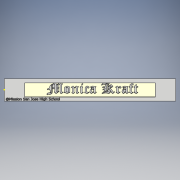
# Autodesk Inventor part: NameTag
Saved by Autodesk Inventor 2018 (Build 220112000, 112)
## iProperties
Created: 2019-03-18
Part Number: NameTag
Material: Generic
Document SubType Name: Modeling
Designer: This kid
Density: 1 g/cm^3
Appearance: Default
Author: This kid
Autodesk Inventor part; units mm, degrees
(part 1 of 3)
ref_plane "YZ Plane" through (0, 0, 0) normal (1, 0, 0) x (0, 1, 0)
ref_plane "XZ Plane" through (0, 0, 0) normal (0, 1, 0) x (-1, 0, 0)
ref_plane "XY Plane" through (0, 0, 0) normal (0, 0, 1) x (1, 0, 0)
sketch "Sketch1" plane through (0, 0, 0) normal (0, 0, 1) x (1, 0, 0)
  line L0 (0, 6.6514) -> (5.7603, -3.3257)
  line L1 (5.7603, -3.3257) -> (-5.7603, -3.3257)
  line L2 (-5.7603, -3.3257) -> (0, 6.6514)
  point P0 (0, 0)
  point P1 (0, 0)
  constraints: 6 end point, 1 coincident, 7 other
extrude "Extrusion1" add sketch "Sketch1" along normal blind 76.2
sketch "Sketch2" plane through (-5.7603, -3.3257, 0) normal (-0.8660254, 0.5, 0) x (0, 0, 1)
  line L0 (9.0292, 2.0917) -> (67.1704, 2.0917)
  line L1 (67.1704, 2.0917) -> (67.1704, 9.2481)
  line L2 (67.1704, 9.2481) -> (9.0292, 9.2481)
  line L3 (9.0292, 9.2481) -> (9.0292, 2.0917)
  line L4 (0, 5.7603) -> (9.0292, 5.6699) construction
  line L5 (67.1704, 5.7603) -> (76.2, 5.7603) construction
  constraints: 12 end point, 2 parallel, 1 equal length, 1 horizontal, 1 midpoint, 1 perpendicular, 1 point on line
extrude "Extrusion2" add sketch "Sketch2" along normal blind 0.2286
sketch "Sketch3" plane through (-5.9582, -3.2114, 0) normal (-0.8660254, 0.5, 0) x (0, 0, 1)
  point P0 (0, 5.7603)
sketch "Sketch4" plane through (-5.9582, -3.2114, 0) normal (-0.8660254, 0.5, 0) x (0, 0, 1)
  line L0 (9.8332, 9.129) -> (68.5929, 9.129) construction
  line L1 (68.5929, 9.129) -> (68.5929, 1.5104) construction
  line L2 (68.5929, 1.5104) -> (9.8332, 1.5104) construction
  line L3 (9.8332, 1.5104) -> (9.8332, 9.129) construction
  line L4 (25.7804, 8.8183) -> (25.8898, 8.7045)
  spline S0 degree 2 poles (25.8898, 8.7045) (25.6535, 8.442) (25.5222, 8.1094) (25.5222, 7.7724) knots 0 0 0 1 2 2 2
  line L5 (25.5222, 7.7724) -> (25.5222, 4.9936)
  spline S1 degree 2 poles (25.5222, 4.9936) (25.5222, 4.5647) (25.6666, 4.3459) (25.7848, 4.3459) knots 0 0 0 1 2 2 2
  spline S2 degree 2 poles (25.7848, 4.3459) (25.8854, 4.3459) (26.0692, 4.5122) knots 0 0 0 1 1 1
  line L6 (26.0692, 4.5122) -> (26.1743, 4.3721)
  line L7 (26.1743, 4.3721) -> (25.3034, 3.6895)
  spline S3 degree 2 poles (25.3034, 3.6895) (24.9883, 3.847) (24.7695, 4.2584) (24.7695, 4.7791) knots 0 0 0 1 2 2 2
  line L8 (24.7695, 4.7791) -> (24.7695, 8.21)
  line L9 (24.7695, 8.21) -> (24.1656, 8.6695)
  line L10 (24.1656, 8.6695) -> (23.9293, 8.5164)
  line L11 (23.9293, 8.5164) -> (23.9293, 6.7396)
  line L12 (23.9293, 6.7396) -> (24.3625, 6.7396)
  line L13 (24.3625, 6.7396) -> (23.9293, 6.2014)
  line L14 (23.9293, 6.2014) -> (23.9293, 4.6872)
  line L15 (23.9293, 4.6872) -> (24.2094, 4.9192)
  line L16 (24.2094, 4.9192) -> (24.3188, 4.8054)
  line L17 (24.3188, 4.8054) -> (22.9928, 3.6895)
  spline S4 degree 2 poles (22.9928, 3.6895) (22.6908, 4.0483) (22.5027, 4.2146) knots 0 0 0 1 1 1
  spline S5 degree 2 poles (22.5027, 4.2146) (22.367, 4.3328) (22.1832, 4.429) knots 0 0 0 1 1 1
  line L18 (22.1832, 4.429) -> (22.1832, 4.5603)
  spline S6 degree 2 poles (22.1832, 4.5603) (22.3539, 4.6172) (22.4064, 4.7441) knots 0 0 0 1 1 1
  spline S7 degree 2 poles (22.4064, 4.7441) (22.4458, 4.836) (22.4458, 5.1817) knots 0 0 0 1 1 1
  line L19 (22.4458, 5.1817) -> (22.4458, 6.2014)
  line L20 (22.4458, 6.2014) -> (21.3561, 6.2014)
  line L21 (21.3561, 6.2014) -> (21.3561, 4.6522)
  spline S8 degree 2 poles (21.3561, 4.6522) (21.3561, 4.0133) (20.7084, 3.3219) (20.1833, 3.3219) knots 0 0 0 1 2 2 2
  spline S9 degree 2 poles (20.1833, 3.3219) (20.0695, 3.3219) (19.7763, 3.3656) knots 0 0 0 1 1 1
  spline S10 degree 2 poles (19.7763, 3.3656) (19.575, 3.3963) (19.4831, 3.3963) knots 0 0 0 1 1 1
  spline S11 degree 2 poles (19.4831, 3.3963) (19.2993, 3.3963) (19.133, 3.23) (19.133, 3.033) knots 0 0 0 1 2 2 2
  line L22 (19.133, 3.033) -> (18.993, 3.033)
  spline S12 degree 2 poles (18.993, 3.033) (18.9492, 3.1862) (18.9492, 3.2912) knots 0 0 0 1 1 1
  spline S13 degree 2 poles (18.9492, 3.2912) (18.9492, 3.4838) (19.1505, 3.8251) (19.3212, 3.9083) knots 0 0 0 1 2 2 2
  spline S14 degree 2 poles (19.3212, 3.9083) (19.4481, 3.9739) (20.1395, 4.0396) (20.4677, 4.4072) (20.4677, 4.7354) knots 0 0 0 1 2 3 3 3
  spline S15 degree 2 poles (20.4677, 4.7354) (20.4677, 5.2474) (19.9864, 5.9126) (19.645, 5.9126) knots 0 0 0 1 2 2 2
  spline S16 degree 2 poles (19.645, 5.9126) (19.3825, 5.9126) (19.2118, 5.6631) knots 0 0 0 1 1 1
  line L23 (19.2118, 5.6631) -> (19.0805, 5.72)
  spline S17 degree 2 poles (19.0805, 5.72) (19.1768, 5.9826) (19.435, 6.267) (19.6494, 6.3502) knots 0 0 0 1 2 2 2
  spline S18 degree 2 poles (19.6494, 6.3502) (19.8069, 6.4114) (20.1089, 6.4158) knots 0 0 0 1 1 1
  spline S19 degree 2 poles (20.1089, 6.4158) (20.1045, 6.5252) (20.1045, 6.5777) knots 0 0 0 1 1 1
  spline S20 degree 2 poles (20.1045, 6.5777) (20.1045, 7.1816) (20.5859, 8.0044) (21.6143, 8.7002) (22.5814, 9.129) knots 0 0 0 1 2 3 3 3
  spline S21 degree 2 poles (22.5814, 9.129) (22.9228, 8.9452) (23.1635, 8.582) (23.1766, 8.2319) knots 0 0 0 1 2 2 2
  line L24 (23.1766, 8.2319) -> (24.5813, 9.129)
  line L25 (24.5813, 9.129) -> (25.4391, 8.4901)
  line L26 (25.4391, 8.4901) -> (25.7804, 8.8183)
  line L27 (22.4458, 6.7396) -> (22.4458, 7.8074)
  spline S22 degree 2 poles (22.4458, 7.8074) (22.4458, 8.2013) (22.2445, 8.5514) (21.9863, 8.6608) knots 0 0 0 1 2 2 2
  spline S23 degree 2 poles (21.9863, 8.6608) (21.7368, 8.5339) (21.6318, 8.4288) knots 0 0 0 1 1 1
  spline S24 degree 2 poles (21.6318, 8.4288) (21.4918, 8.2801) (21.3561, 7.8731) (21.3561, 7.488) knots 0 0 0 1 2 2 2
  line L28 (21.3561, 7.488) -> (21.3561, 6.3502)
  line L29 (21.3561, 6.3502) -> (21.6537, 6.7396)
  line L30 (21.6537, 6.7396) -> (22.4458, 6.7396)
  spline S25 degree 2 poles (21.3299, 8.2801) (21.0191, 8.0394) (20.8353, 7.5974) (20.8353, 7.046) knots 0 0 0 1 2 2 2
  line L31 (20.8353, 7.046) -> (20.8353, 5.0111)
  spline S26 degree 2 poles (20.8353, 5.0111) (20.8353, 4.5122) (20.5815, 4.1096) (20.2139, 3.9608) knots 0 0 0 1 2 2 2
  spline S27 degree 2 poles (20.2139, 3.9608) (20.3758, 3.952) (20.4896, 3.952) knots 0 0 0 1 1 1
  spline S28 degree 2 poles (20.4896, 3.952) (20.7522, 3.952) (21.0848, 4.1358) (21.1898, 4.4028) (21.1898, 4.7441) knots 0 0 0 1 2 3 3 3
  line L32 (21.1898, 4.7441) -> (21.1898, 7.453)
  spline S29 degree 2 poles (21.1898, 7.453) (21.1898, 7.7593) (21.2292, 7.965) knots 0 0 0 1 1 1
  spline S30 degree 2 poles (21.2292, 7.965) (21.2511, 8.0919) (21.3299, 8.2801) knots 0 0 0 1 1 1
  line L33 (23.7718, 6.2014) -> (23.1766, 6.2014)
  line L34 (23.1766, 6.2014) -> (23.1766, 5.2693)
  spline S31 degree 2 poles (23.1766, 5.2693) (23.1766, 4.7879) (23.2422, 4.6522) knots 0 0 0 1 1 1
  spline S32 degree 2 poles (23.2422, 4.6522) (23.3473, 4.4159) (23.5223, 4.4159) knots 0 0 0 1 1 1
  spline S33 degree 2 poles (23.5223, 4.4159) (23.6142, 4.4159) (23.7718, 4.5559) knots 0 0 0 1 1 1
  line L35 (23.7718, 4.5559) -> (23.7718, 6.2014)
  line L36 (23.7718, 8.4157) -> (23.1766, 8.0262)
  line L37 (23.1766, 8.0262) -> (23.1766, 6.7396)
  line L38 (23.1766, 6.7396) -> (23.7718, 6.7396)
  line L39 (23.7718, 6.7396) -> (23.7718, 8.4157)
  line L40 (29.1457, 6.9935) -> (29.1457, 4.3065)
  spline S34 degree 2 poles (29.1457, 4.3065) (28.603, 4.0877) (28.3624, 3.9477) knots 0 0 0 1 1 1
  spline S35 degree 2 poles (28.3624, 3.9477) (28.1786, 3.8426) (28.0123, 3.6895) knots 0 0 0 1 1 1
  spline S36 degree 2 poles (28.0123, 3.6895) (27.4915, 4.0045) (27.1502, 4.1271) knots 0 0 0 1 1 1
  spline S37 degree 2 poles (27.1502, 4.1271) (26.892, 4.219) (26.5637, 4.2321) knots 0 0 0 1 1 1
  line L41 (26.5637, 4.2321) -> (26.5287, 4.3021)
  spline S38 degree 2 poles (26.5287, 4.3021) (26.6644, 4.4159) (26.6994, 4.5122) knots 0 0 0 1 1 1
  spline S39 degree 2 poles (26.6994, 4.5122) (26.7519, 4.6347) (26.7519, 4.9235) knots 0 0 0 1 1 1
  line L42 (26.7519, 4.9235) -> (26.7519, 6.9016)
  spline S40 degree 2 poles (26.7519, 6.9016) (27.4127, 7.1204) (27.881, 7.5186) knots 0 0 0 1 1 1
  spline S41 degree 2 poles (27.881, 7.5186) (28.3886, 7.1816) (29.1457, 6.9935) knots 0 0 0 1 1 1
  line L43 (27.4784, 4.6566) -> (28.4149, 4.2715)
  line L44 (28.4149, 4.2715) -> (28.4149, 6.5515)
  spline S42 degree 2 poles (28.4149, 6.5515) (27.9729, 6.7615) (27.7891, 6.8272) knots 0 0 0 1 1 1
  spline S43 degree 2 poles (27.7891, 6.8272) (27.6622, 6.8709) (27.4784, 6.9059) knots 0 0 0 1 1 1
  line L45 (27.4784, 6.9059) -> (27.4784, 4.6566)
  line L46 (32.0865, 7.5186) -> (32.5766, 6.9803)
  line L47 (32.5766, 6.9803) -> (32.9267, 7.3173)
  line L48 (32.9267, 7.3173) -> (33.023, 7.221)
  spline S44 degree 2 poles (33.023, 7.221) (32.7735, 6.9891) (32.7166, 6.8709) knots 0 0 0 1 1 1
  spline S45 degree 2 poles (32.7166, 6.8709) (32.6466, 6.7134) (32.6466, 6.4333) knots 0 0 0 1 1 1
  line L49 (32.6466, 6.4333) -> (32.6466, 4.7222)
  spline S46 degree 2 poles (32.6466, 4.7222) (32.6466, 4.4859) (32.721, 4.3678) knots 0 0 0 1 1 1
  spline S47 degree 2 poles (32.721, 4.3678) (32.7692, 4.2934) (32.826, 4.2934) knots 0 0 0 1 1 1
  spline S48 degree 2 poles (32.826, 4.2934) (32.8786, 4.2934) (33.0667, 4.429) knots 0 0 0 1 1 1
  line L50 (33.0667, 4.429) -> (33.1499, 4.3196)
  line L51 (33.1499, 4.3196) -> (32.384, 3.6895)
  spline S49 degree 2 poles (32.384, 3.6895) (32.0865, 3.9126) (31.9158, 4.2584) (31.9158, 4.6478) knots 0 0 0 1 2 2 2
  line L52 (31.9158, 4.6478) -> (31.9158, 6.6127)
  line L53 (31.9158, 6.6127) -> (31.5963, 6.9453)
  line L54 (31.5963, 6.9453) -> (30.9837, 6.4552)
  line L55 (30.9837, 6.4552) -> (30.9837, 4.464)
  line L56 (30.9837, 4.464) -> (31.255, 4.2058)
  line L57 (31.255, 4.2058) -> (30.6205, 3.6895)
  line L58 (30.6205, 3.6895) -> (29.9815, 4.2058)
  line L59 (29.9815, 4.2058) -> (30.2529, 4.464)
  line L60 (30.2529, 4.464) -> (30.2529, 6.2933)
  spline S50 degree 2 poles (30.2529, 6.2933) (30.2529, 6.6871) (30.1741, 6.8228) knots 0 0 0 1 1 1
  spline S51 degree 2 poles (30.1741, 6.8228) (30.1216, 6.9147) (30.0516, 6.9147) knots 0 0 0 1 1 1
  spline S52 degree 2 poles (30.0516, 6.9147) (29.9772, 6.9147) (29.8371, 6.779) knots 0 0 0 1 1 1
  line L61 (29.8371, 6.779) -> (29.7496, 6.8884)
  line L62 (29.7496, 6.8884) -> (30.511, 7.5186)
  spline S53 degree 2 poles (30.511, 7.5186) (30.8261, 7.2823) (30.9837, 7.0066) (30.9837, 6.7659) knots 0 0 0 1 2 2 2
  line L63 (30.9837, 6.7659) -> (30.9837, 6.6346)
  line L64 (30.9837, 6.6346) -> (32.0865, 7.5186)
  line L65 (34.2702, 7.5186) -> (34.9047, 6.9935)
  line L66 (34.9047, 6.9935) -> (34.6203, 6.7134)
  line L67 (34.6203, 6.7134) -> (34.6203, 4.7572)
  spline S54 degree 2 poles (34.6203, 4.7572) (34.6203, 4.4509) (34.7253, 4.2627) (34.7778, 4.2627) knots 0 0 0 1 2 2 2
  spline S55 degree 2 poles (34.7778, 4.2627) (34.8172, 4.2627) (34.8522, 4.2802) knots 0 0 0 1 1 1
  spline S56 degree 2 poles (34.8522, 4.2802) (34.896, 4.3065) (35.0404, 4.429) knots 0 0 0 1 1 1
  line L68 (35.0404, 4.429) -> (35.1235, 4.3196)
  line L69 (35.1235, 4.3196) -> (34.3577, 3.6895)
  spline S57 degree 2 poles (34.3577, 3.6895) (34.0689, 3.8951) (33.9026, 4.2584) (33.9026, 4.7091) knots 0 0 0 1 2 2 2
  line L70 (33.9026, 4.7091) -> (33.9026, 6.7134)
  line L71 (33.9026, 6.7134) -> (33.6313, 6.9935)
  line L72 (33.6313, 6.9935) -> (34.2702, 7.5186)
  line L73 (34.5371, 8.7439) -> (34.9922, 8.7439)
  line L74 (34.9922, 8.7439) -> (34.4977, 7.9693)
  line L75 (34.4977, 7.9693) -> (34.3533, 7.9693)
  line L76 (34.3533, 7.9693) -> (34.5371, 8.7439)
  line L77 (36.8127, 7.5186) -> (37.7449, 6.9891)
  line L78 (37.7449, 6.9891) -> (37.3685, 6.4246)
  line L79 (37.3685, 6.4246) -> (36.6596, 6.8315)
  line L80 (36.6596, 6.8315) -> (36.6596, 4.5384)
  line L81 (36.6596, 4.5384) -> (37.3641, 4.2234)
  line L82 (37.3641, 4.2234) -> (37.7405, 4.5034)
  line L83 (37.7405, 4.5034) -> (37.7799, 4.3459)
  line L84 (37.7799, 4.3459) -> (36.8915, 3.6895)
  spline S58 degree 2 poles (36.8915, 3.6895) (36.5458, 3.882) (36.06, 4.0658) (35.7056, 4.1358) knots 0 0 0 1 2 2 2
  line L85 (35.7056, 4.1358) -> (35.7056, 4.2234)
  spline S59 degree 2 poles (35.7056, 4.2234) (35.8325, 4.3109) (35.8719, 4.4115) knots 0 0 0 1 1 1
  spline S60 degree 2 poles (35.8719, 4.4115) (35.9287, 4.5516) (35.9287, 4.8491) knots 0 0 0 1 1 1
  line L86 (35.9287, 4.8491) -> (35.9287, 6.8884)
  spline S61 degree 2 poles (35.9287, 6.8884) (36.3751, 7.0941) (36.8127, 7.5186) knots 0 0 0 1 1 1
  line L87 (40.6594, 7.3654) -> (40.7907, 7.3173)
  spline S62 degree 2 poles (40.7907, 7.3173) (40.5937, 7.0153) (40.4887, 6.6959) (40.4887, 6.4202) knots 0 0 0 1 2 2 2
  line L88 (40.4887, 6.4202) -> (40.4887, 4.8929)
  spline S63 degree 2 poles (40.4887, 4.8929) (40.4887, 4.5122) (40.5981, 4.3196) (40.6725, 4.3196) knots 0 0 0 1 2 2 2
  spline S64 degree 2 poles (40.6725, 4.3196) (40.7119, 4.3196) (40.7513, 4.3415) knots 0 0 0 1 1 1
  spline S65 degree 2 poles (40.7513, 4.3415) (40.7775, 4.3546) (40.9088, 4.4597) knots 0 0 0 1 1 1
  line L89 (40.9088, 4.4597) -> (40.992, 4.3503)
  line L90 (40.992, 4.3503) -> (40.2349, 3.6895)
  spline S66 degree 2 poles (40.2349, 3.6895) (39.9548, 3.9039) (39.7666, 4.2452) (39.7579, 4.5516) knots 0 0 0 1 2 2 2
  line L91 (39.7579, 4.5516) -> (38.6682, 3.6895)
  spline S67 degree 2 poles (38.6682, 3.6895) (38.0512, 4.1927) (38.0512, 4.6828) knots 0 0 0 1 1 1
  spline S68 degree 2 poles (38.0512, 4.6828) (38.0512, 5.0111) (38.1825, 5.2999) knots 0 0 0 1 1 1
  spline S69 degree 2 poles (38.1825, 5.2999) (38.3619, 5.6762) (38.7951, 6.1795) knots 0 0 0 1 1 1
  line L92 (38.7951, 6.1795) -> (38.3575, 7.0985)
  line L93 (38.3575, 7.0985) -> (38.41, 7.1948)
  spline S70 degree 2 poles (38.41, 7.1948) (38.5501, 7.186) (38.6201, 7.186) knots 0 0 0 1 1 1
  spline S71 degree 2 poles (38.6201, 7.186) (39.0402, 7.186) (39.364, 7.5186) knots 0 0 0 1 1 1
  spline S72 degree 2 poles (39.364, 7.5186) (39.6266, 7.3654) (40.248, 7.1816) (40.4099, 7.1816) knots 0 0 0 1 2 2 2
  spline S73 degree 2 poles (40.4099, 7.1816) (40.4887, 7.1816) (40.5675, 7.2342) (40.6594, 7.3654) knots 0 0 0 1 2 2 2
  line L94 (39.7579, 5.6106) -> (38.887, 6.022)
  spline S74 degree 2 poles (38.887, 6.022) (38.6857, 5.58) (38.6857, 5.2518) knots 0 0 0 1 1 1
  spline S75 degree 2 poles (38.6857, 5.2518) (38.6857, 4.6697) (39.2109, 4.2934) knots 0 0 0 1 1 1
  line L95 (39.2109, 4.2934) -> (39.7579, 4.7266)
  line L96 (39.7579, 4.7266) -> (39.7579, 5.6106)
  line L97 (39.7579, 6.6828) -> (38.5282, 7.0591)
  line L98 (38.5282, 7.0591) -> (38.9658, 6.1314)
  line L99 (38.9658, 6.1314) -> (39.7579, 5.7594)
  line L100 (39.7579, 5.7594) -> (39.7579, 6.6828)
  line L101 (46.5978, 9.129) -> (46.7335, 9.0503)
  spline S76 degree 2 poles (46.7335, 9.0503) (46.4315, 8.5383) (46.1777, 7.7549) (46.1383, 7.2298) knots 0 0 0 1 2 2 2
  line L102 (46.1383, 7.2298) -> (47.5168, 8.3194)
  line L103 (47.5168, 8.3194) -> (48.3527, 7.3479)
  line L104 (48.3527, 7.3479) -> (46.9217, 6.3327)
  spline S77 degree 2 poles (46.9217, 6.3327) (47.2499, 6.1532) (47.7444, 5.6325) (48.3964, 4.5253) (48.5409, 4.3721) (48.6065, 4.3721) knots 0 0 0 1 2 3 4 4 4
  spline S78 degree 2 poles (48.6065, 4.3721) (48.6765, 4.3721) (48.8166, 4.5122) knots 0 0 0 1 1 1
  line L105 (48.8166, 4.5122) -> (49.0047, 4.6872)
  line L106 (49.0047, 4.6872) -> (49.1141, 4.5559)
  line L107 (49.1141, 4.5559) -> (48.2214, 3.6895)
  spline S79 degree 2 poles (48.2214, 3.6895) (48.0332, 3.8207) (47.8188, 4.0964) (47.4556, 4.7485) knots 0 0 0 1 2 2 2
  line L108 (47.4556, 4.7485) -> (46.5278, 3.6895)
  spline S80 degree 2 poles (46.5278, 3.6895) (46.099, 3.8776) (45.4031, 4.0439) (45.0355, 4.0439) knots 0 0 0 1 2 2 2
  spline S81 degree 2 poles (45.0355, 4.0439) (44.6767, 4.0439) (43.9896, 3.882) (43.5433, 3.6895) knots 0 0 0 1 2 2 2
  line L109 (43.5433, 3.6895) -> (43.4251, 3.8558)
  spline S82 degree 2 poles (43.4251, 3.8558) (44.1297, 4.4159) (44.436, 4.8491) knots 0 0 0 1 1 1
  spline S83 degree 2 poles (44.436, 4.8491) (44.5848, 5.0636) (44.5848, 5.2649) knots 0 0 0 1 1 1
  spline S84 degree 2 poles (44.5848, 5.2649) (44.5848, 5.4574) (44.331, 5.7069) (44.1603, 5.7069) knots 0 0 0 1 2 2 2
  spline S85 degree 2 poles (44.1603, 5.7069) (44.0028, 5.7069) (43.8802, 5.5493) knots 0 0 0 1 1 1
  line L110 (43.8802, 5.5493) -> (43.7533, 5.6106)
  spline S86 degree 2 poles (43.7533, 5.6106) (43.819, 5.8207) (44.1253, 6.0526) (44.3179, 6.0526) knots 0 0 0 1 2 2 2
  spline S87 degree 2 poles (44.3179, 6.0526) (44.4448, 6.0526) (44.7161, 5.9519) (44.8649, 5.8469) knots 0 0 0 1 2 2 2
  spline S88 degree 2 poles (44.8649, 5.8469) (44.8736, 5.9651) (44.8736, 6.0482) knots 0 0 0 1 1 1
  spline S89 degree 2 poles (44.8736, 6.0482) (44.8736, 6.4333) (44.4273, 6.9059) (44.1166, 6.9059) knots 0 0 0 1 2 2 2
  spline S90 degree 2 poles (44.1166, 6.9059) (43.9371, 6.9059) (43.7577, 6.7484) knots 0 0 0 1 1 1
  line L111 (43.7577, 6.7484) -> (43.6352, 6.7965)
  spline S91 degree 2 poles (43.6352, 6.7965) (43.7227, 7.0241) (44.0597, 7.256) (44.2828, 7.256) knots 0 0 0 1 2 2 2
  spline S92 degree 2 poles (44.2828, 7.256) (44.401, 7.256) (44.6811, 7.1598) (44.8342, 7.0635) knots 0 0 0 1 2 2 2
  spline S93 degree 2 poles (44.8342, 7.0635) (44.8255, 7.2123) (44.8255, 7.3261) knots 0 0 0 1 1 1
  spline S94 degree 2 poles (44.8255, 7.3261) (44.8255, 7.6586) (45.1012, 8.1663) (45.7445, 8.8402) knots 0 0 0 1 2 2 2
  spline S95 degree 2 poles (45.7445, 8.8402) (45.3638, 8.6214) (44.9218, 8.4726) (44.703, 8.4726) knots 0 0 0 1 2 2 2
  spline S96 degree 2 poles (44.703, 8.4726) (44.5892, 8.4726) (44.2216, 8.5383) (44.1428, 8.5383) knots 0 0 0 1 2 2 2
  spline S97 degree 2 poles (44.1428, 8.5383) (43.8802, 8.5383) (43.517, 8.2713) (43.3551, 7.9562) knots 0 0 0 1 2 2 2
  line L112 (43.3551, 7.9562) -> (43.2326, 7.9825)
  spline S98 degree 2 poles (43.2326, 7.9825) (43.307, 8.3457) (43.4164, 8.5251) knots 0 0 0 1 1 1
  spline S99 degree 2 poles (43.4164, 8.5251) (43.587, 8.814) (44.0903, 9.129) (44.3529, 9.129) knots 0 0 0 1 2 2 2
  spline S100 degree 2 poles (44.3529, 9.129) (44.5542, 9.129) (45.1493, 8.9409) (45.3419, 8.9409) knots 0 0 0 1 2 2 2
  spline S101 degree 2 poles (45.3419, 8.9409) (45.6526, 8.9409) (46.0158, 9.129) knots 0 0 0 1 1 1
  line L113 (46.0158, 9.129) -> (46.1427, 9.0503)
  spline S102 degree 2 poles (46.1427, 9.0503) (45.8451, 8.617) (45.5476, 7.5055) (45.5476, 6.9847) knots 0 0 0 1 2 2 2
  line L114 (45.5476, 6.9847) -> (45.5607, 5.9607)
  spline S103 degree 2 poles (45.5607, 5.9607) (45.5607, 5.7331) (45.4163, 5.348) (45.1493, 5.0417) (45.1143, 5.0154) knots 0 0 0 1 2 3 3 3
  line L115 (45.1143, 5.0154) -> (44.0597, 4.1315)
  spline S104 degree 2 poles (44.0597, 4.1315) (44.3397, 4.2802) (44.6548, 4.4159) knots 0 0 0 1 1 1
  spline S105 degree 2 poles (44.6548, 4.4159) (45.2281, 4.661) (45.7182, 5.0198) (45.9852, 5.5756) (45.9852, 6.0001) knots 0 0 0 1 2 3 3 3
  line L116 (45.9852, 6.0001) -> (45.972, 7.1204)
  spline S106 degree 2 poles (45.972, 7.1204) (45.972, 7.523) (46.2521, 8.5601) (46.5978, 9.129) knots 0 0 0 1 2 2 2
  spline S107 degree 2 poles (47.3724, 4.8885) (47.0398, 5.4224) (46.4753, 5.8207) (46.1383, 5.8338) knots 0 0 0 1 2 2 2
  spline S108 degree 2 poles (46.1383, 5.8338) (46.1296, 5.4268) (45.8276, 4.8885) (45.4775, 4.6435) knots 0 0 0 1 2 2 2
  spline S109 degree 2 poles (45.4775, 4.6435) (46.0289, 4.6128) (46.5541, 4.4859) (46.8735, 4.3196) knots 0 0 0 1 2 2 2
  line L117 (46.8735, 4.3196) -> (47.3724, 4.8885)
  line L118 (47.0486, 7.7462) -> (46.1383, 7.0197)
  line L119 (46.1383, 7.0197) -> (46.1383, 6.9103)
  line L120 (46.1383, 6.9103) -> (46.1471, 6.3414)
  line L121 (46.1471, 6.3414) -> (46.1383, 5.9913)
  line L122 (46.1383, 5.9913) -> (47.6481, 7.0547)
  line L123 (47.6481, 7.0547) -> (47.0486, 7.7462)
  line L124 (51.4729, 7.5186) -> (52.0112, 6.8709)
  line L125 (52.0112, 6.8709) -> (51.4729, 6.3896)
  line L126 (51.4729, 6.3896) -> (51.0178, 6.9585)
  line L127 (51.0178, 6.9585) -> (50.6633, 6.6346)
  line L128 (50.6633, 6.6346) -> (50.6633, 4.5428)
  line L129 (50.6633, 4.5428) -> (51.0747, 4.2496)
  line L130 (51.0747, 4.2496) -> (51.4423, 4.5341)
  line L131 (51.4423, 4.5341) -> (51.5254, 4.4247)
  line L132 (51.5254, 4.4247) -> (50.6064, 3.6895)
  spline S110 degree 2 poles (50.6064, 3.6895) (50.3132, 3.952) (49.915, 4.1796) (49.6787, 4.2452) knots 0 0 0 1 2 2 2
  line L133 (49.6787, 4.2452) -> (49.6787, 4.324)
  spline S111 degree 2 poles (49.6787, 4.324) (49.8362, 4.4334) (49.9325, 4.661) (49.9325, 4.9804) knots 0 0 0 1 2 2 2
  line L134 (49.9325, 4.9804) -> (49.9325, 6.4508)
  spline S112 degree 2 poles (49.9325, 6.4508) (49.9325, 6.7265) (49.8099, 6.9103) (49.7355, 6.9103) knots 0 0 0 1 2 2 2
  spline S113 degree 2 poles (49.7355, 6.9103) (49.6568, 6.9103) (49.5167, 6.7615) knots 0 0 0 1 1 1
  line L135 (49.5167, 6.7615) -> (49.4292, 6.8709)
  line L136 (49.4292, 6.8709) -> (50.1775, 7.5186)
  spline S114 degree 2 poles (50.1775, 7.5186) (50.4795, 7.2867) (50.5933, 7.1116) knots 0 0 0 1 1 1
  spline S115 degree 2 poles (50.5933, 7.1116) (50.6633, 7.0066) (50.6633, 6.814) knots 0 0 0 1 1 1
  line L137 (50.6633, 6.814) -> (51.4729, 7.5186)
  line L138 (54.9476, 7.3654) -> (55.0788, 7.3173)
  spline S116 degree 2 poles (55.0788, 7.3173) (54.8819, 7.0153) (54.7769, 6.6959) (54.7769, 6.4202) knots 0 0 0 1 2 2 2
  line L139 (54.7769, 6.4202) -> (54.7769, 4.8929)
  spline S117 degree 2 poles (54.7769, 4.8929) (54.7769, 4.5122) (54.8863, 4.3196) (54.9607, 4.3196) knots 0 0 0 1 2 2 2
  spline S118 degree 2 poles (54.9607, 4.3196) (55.0001, 4.3196) (55.0395, 4.3415) knots 0 0 0 1 1 1
  spline S119 degree 2 poles (55.0395, 4.3415) (55.0657, 4.3546) (55.197, 4.4597) knots 0 0 0 1 1 1
  line L140 (55.197, 4.4597) -> (55.2802, 4.3503)
  line L141 (55.2802, 4.3503) -> (54.5231, 3.6895)
  spline S120 degree 2 poles (54.5231, 3.6895) (54.243, 3.9039) (54.0548, 4.2452) (54.0461, 4.5516) knots 0 0 0 1 2 2 2
  line L142 (54.0461, 4.5516) -> (52.9564, 3.6895)
  spline S121 degree 2 poles (52.9564, 3.6895) (52.3394, 4.1927) (52.3394, 4.6828) knots 0 0 0 1 1 1
  spline S122 degree 2 poles (52.3394, 4.6828) (52.3394, 5.0111) (52.4707, 5.2999) knots 0 0 0 1 1 1
  spline S123 degree 2 poles (52.4707, 5.2999) (52.6501, 5.6762) (53.0833, 6.1795) knots 0 0 0 1 1 1
  line L143 (53.0833, 6.1795) -> (52.6457, 7.0985)
  line L144 (52.6457, 7.0985) -> (52.6982, 7.1948)
  spline S124 degree 2 poles (52.6982, 7.1948) (52.8383, 7.186) (52.9083, 7.186) knots 0 0 0 1 1 1
  spline S125 degree 2 poles (52.9083, 7.186) (53.3284, 7.186) (53.6522, 7.5186) knots 0 0 0 1 1 1
  spline S126 degree 2 poles (53.6522, 7.5186) (53.9148, 7.3654) (54.5362, 7.1816) (54.6981, 7.1816) knots 0 0 0 1 2 2 2
  spline S127 degree 2 poles (54.6981, 7.1816) (54.7769, 7.1816) (54.8557, 7.2342) (54.9476, 7.3654) knots 0 0 0 1 2 2 2
  line L145 (54.0461, 5.6106) -> (53.1752, 6.022)
  spline S128 degree 2 poles (53.1752, 6.022) (52.9739, 5.58) (52.9739, 5.2518) knots 0 0 0 1 1 1
  spline S129 degree 2 poles (52.9739, 5.2518) (52.9739, 4.6697) (53.4991, 4.2934) knots 0 0 0 1 1 1
  line L146 (53.4991, 4.2934) -> (54.0461, 4.7266)
  line L147 (54.0461, 4.7266) -> (54.0461, 5.6106)
  line L148 (54.0461, 6.6828) -> (52.8164, 7.0591)
  line L149 (52.8164, 7.0591) -> (53.254, 6.1314)
  line L150 (53.254, 6.1314) -> (54.0461, 5.7594)
  line L151 (54.0461, 5.7594) -> (54.0461, 6.6828)
  line L152 (57.3851, 8.6652) -> (57.2757, 8.07)
  line L153 (57.2757, 8.07) -> (56.6193, 8.2188)
  line L154 (56.6193, 8.2188) -> (56.6193, 7.3523)
  line L155 (56.6193, 7.3523) -> (57.175, 7.3523)
  line L156 (57.175, 7.3523) -> (57.175, 6.9497)
  line L157 (57.175, 6.9497) -> (56.6193, 6.9497)
  line L158 (56.6193, 6.9497) -> (56.6193, 4.5428)
  line L159 (56.6193, 4.5428) -> (57.0262, 4.2365)
  line L160 (57.0262, 4.2365) -> (57.3063, 4.4597)
  line L161 (57.3063, 4.4597) -> (57.3895, 4.359)
  line L162 (57.3895, 4.359) -> (56.558, 3.6895)
  spline S130 degree 2 poles (56.558, 3.6895) (56.1116, 4.0877) (55.6434, 4.2321) knots 0 0 0 1 1 1
  line L163 (55.6434, 4.2321) -> (55.6215, 4.3196)
  spline S131 degree 2 poles (55.6215, 4.3196) (55.7528, 4.4028) (55.8009, 4.4903) knots 0 0 0 1 1 1
  spline S132 degree 2 poles (55.8009, 4.4903) (55.8884, 4.6391) (55.8884, 4.8491) knots 0 0 0 1 1 1
  line L164 (55.8884, 4.8491) -> (55.8884, 6.9497)
  line L165 (55.8884, 6.9497) -> (55.5515, 6.9497)
  line L166 (55.5515, 6.9497) -> (55.5515, 7.3523)
  line L167 (55.5515, 7.3523) -> (55.8884, 7.3523)
  line L168 (55.8884, 7.3523) -> (55.8884, 8.2188)
  spline S133 degree 2 poles (55.8884, 8.2188) (56.4267, 8.5864) (56.7024, 8.8358) knots 0 0 0 1 1 1
  line L169 (56.7024, 8.8358) -> (57.3851, 8.6652)
  line L170 (57.6477, 7.1247) -> (58.6454, 8.3588)
  line L171 (58.6454, 8.3588) -> (58.7505, 8.3588)
  line L172 (58.7505, 8.3588) -> (58.7154, 7.3698)
  line L173 (58.7154, 7.3698) -> (59.4375, 7.3698)
  line L174 (59.4375, 7.3698) -> (59.4375, 6.9672)
  line L175 (59.4375, 6.9672) -> (58.7154, 6.9672)
  line L176 (58.7154, 6.9672) -> (58.7154, 4.5472)
  line L177 (58.7154, 4.5472) -> (59.1181, 4.2496)
  line L178 (59.1181, 4.2496) -> (59.35, 4.429)
  line L179 (59.35, 4.429) -> (59.4419, 4.3196)
  line L180 (59.4419, 4.3196) -> (58.6498, 3.6895)
  spline S134 degree 2 poles (58.6498, 3.6895) (58.2428, 4.1008) (57.7352, 4.2496) knots 0 0 0 1 1 1
  line L181 (57.7352, 4.2496) -> (57.7352, 4.3196)
  spline S135 degree 2 poles (57.7352, 4.3196) (57.8796, 4.4159) (57.9234, 4.5209) knots 0 0 0 1 1 1
  spline S136 degree 2 poles (57.9234, 4.5209) (57.9846, 4.6522) (57.9846, 4.906) knots 0 0 0 1 1 1
  line L182 (57.9846, 4.906) -> (57.9846, 6.9672)
  line L183 (57.9846, 6.9672) -> (57.6477, 6.9672)
  line L184 (57.6477, 6.9672) -> (57.6477, 7.1247)
  point P0 (0, 5.7603)
  constraints: 2 other
extrude "Extrusion3" add sketch "Sketch4" along normal blind 0.254
sketch "Sketch5" plane through (0, 6.6514, 76.2) normal (0.8660254, 0.5, 0) x (0, 0, -1)
  line L0 (67.0697, -2.2328) -> (67.0697, -9.3892)
  line L1 (9.3366, -9.3892) -> (67.0697, -9.3892)
  line L2 (67.0697, -2.2328) -> (9.3366, -2.2328)
  line L3 (9.3366, -2.2328) -> (9.3366, -9.3892)
  line L4 (67.0697, -5.811) -> (76.4063, -5.811) construction
  line L5 (0, -5.7603) -> (9.3366, -5.7603) construction
  constraints: 12 end point, 1 horizontal, 1 midpoint, 1 parallel, 1 perpendicular, 1 point on line, 1 vertical
extrude "Extrusion4" add sketch "Sketch5" along normal blind 0.2286
sketch "Sketch6" plane through (0.198, 6.7657, 76.2) normal (0.8660254, 0.5, 0) x (0, 0, -1)
  line L0 (12.3096, -2.534) -> (68.3434, -2.534) construction
  line L1 (68.3434, -2.534) -> (68.3434, -8.4681) construction
  line L2 (68.3434, -8.4681) -> (12.3096, -8.4681) construction
  line L3 (12.3096, -8.4681) -> (12.3096, -2.534) construction
  line L4 (26.8939, -2.8447) -> (27.0033, -2.9585)
  spline S0 degree 2 poles (27.0033, -2.9585) (26.767, -3.2211) (26.6357, -3.5537) (26.6357, -3.8906) knots 0 0 0 1 2 2 2
  line L5 (26.6357, -3.8906) -> (26.6357, -6.6695)
  spline S1 degree 2 poles (26.6357, -6.6695) (26.6357, -7.0984) (26.7801, -7.3172) (26.8982, -7.3172) knots 0 0 0 1 2 2 2
  spline S2 degree 2 poles (26.8982, -7.3172) (26.9989, -7.3172) (27.1827, -7.1509) knots 0 0 0 1 1 1
  line L6 (27.1827, -7.1509) -> (27.2877, -7.2909)
  line L7 (27.2877, -7.2909) -> (26.4169, -7.9736)
  spline S3 degree 2 poles (26.4169, -7.9736) (26.1018, -7.816) (25.883, -7.4047) (25.883, -6.8839) knots 0 0 0 1 2 2 2
  line L8 (25.883, -6.8839) -> (25.883, -3.453)
  line L9 (25.883, -3.453) -> (25.2791, -2.9935)
  line L10 (25.2791, -2.9935) -> (25.0428, -3.1467)
  line L11 (25.0428, -3.1467) -> (25.0428, -4.9234)
  line L12 (25.0428, -4.9234) -> (25.476, -4.9234)
  line L13 (25.476, -4.9234) -> (25.0428, -5.4617)
  line L14 (25.0428, -5.4617) -> (25.0428, -6.9758)
  line L15 (25.0428, -6.9758) -> (25.3228, -6.7439)
  line L16 (25.3228, -6.7439) -> (25.4322, -6.8577)
  line L17 (25.4322, -6.8577) -> (24.1063, -7.9736)
  spline S4 degree 2 poles (24.1063, -7.9736) (23.8043, -7.6147) (23.6161, -7.4484) knots 0 0 0 1 1 1
  spline S5 degree 2 poles (23.6161, -7.4484) (23.4805, -7.3303) (23.2967, -7.234) knots 0 0 0 1 1 1
  line L18 (23.2967, -7.234) -> (23.2967, -7.1027)
  spline S6 degree 2 poles (23.2967, -7.1027) (23.4673, -7.0458) (23.5198, -6.9189) knots 0 0 0 1 1 1
  spline S7 degree 2 poles (23.5198, -6.9189) (23.5592, -6.827) (23.5592, -6.4813) knots 0 0 0 1 1 1
  line L19 (23.5592, -6.4813) -> (23.5592, -5.4617)
  line L20 (23.5592, -5.4617) -> (22.4696, -5.4617)
  line L21 (22.4696, -5.4617) -> (22.4696, -7.0108)
  spline S8 degree 2 poles (22.4696, -7.0108) (22.4696, -7.6497) (21.8219, -8.3412) (21.2968, -8.3412) knots 0 0 0 1 2 2 2
  spline S9 degree 2 poles (21.2968, -8.3412) (21.183, -8.3412) (20.8898, -8.2974) knots 0 0 0 1 1 1
  spline S10 degree 2 poles (20.8898, -8.2974) (20.6885, -8.2668) (20.5966, -8.2668) knots 0 0 0 1 1 1
  spline S11 degree 2 poles (20.5966, -8.2668) (20.4128, -8.2668) (20.2465, -8.4331) (20.2465, -8.63) knots 0 0 0 1 2 2 2
  line L22 (20.2465, -8.63) -> (20.1064, -8.63)
  spline S12 degree 2 poles (20.1064, -8.63) (20.0627, -8.4768) (20.0627, -8.3718) knots 0 0 0 1 1 1
  spline S13 degree 2 poles (20.0627, -8.3718) (20.0627, -8.1793) (20.264, -7.8379) (20.4347, -7.7548) knots 0 0 0 1 2 2 2
  spline S14 degree 2 poles (20.4347, -7.7548) (20.5616, -7.6891) (21.253, -7.6235) (21.5812, -7.2559) (21.5812, -6.9277) knots 0 0 0 1 2 3 3 3
  spline S15 degree 2 poles (21.5812, -6.9277) (21.5812, -6.4157) (21.0998, -5.7505) (20.7585, -5.7505) knots 0 0 0 1 2 2 2
  spline S16 degree 2 poles (20.7585, -5.7505) (20.4959, -5.7505) (20.3252, -5.9999) knots 0 0 0 1 1 1
  line L23 (20.3252, -5.9999) -> (20.194, -5.943)
  spline S17 degree 2 poles (20.194, -5.943) (20.2902, -5.6805) (20.5484, -5.396) (20.7629, -5.3129) knots 0 0 0 1 2 2 2
  spline S18 degree 2 poles (20.7629, -5.3129) (20.9204, -5.2516) (21.2224, -5.2472) knots 0 0 0 1 1 1
  spline S19 degree 2 poles (21.2224, -5.2472) (21.218, -5.1378) (21.218, -5.0853) knots 0 0 0 1 1 1
  spline S20 degree 2 poles (21.218, -5.0853) (21.218, -4.4814) (21.6994, -3.6587) (22.7278, -2.9629) (23.6949, -2.534) knots 0 0 0 1 2 3 3 3
  spline S21 degree 2 poles (23.6949, -2.534) (24.0362, -2.7178) (24.2769, -3.081) (24.2901, -3.4311) knots 0 0 0 1 2 2 2
  line L24 (24.2901, -3.4311) -> (25.6948, -2.534)
  line L25 (25.6948, -2.534) -> (26.5525, -3.1729)
  line L26 (26.5525, -3.1729) -> (26.8939, -2.8447)
  line L27 (23.5592, -4.9234) -> (23.5592, -3.8556)
  spline S22 degree 2 poles (23.5592, -3.8556) (23.5592, -3.4618) (23.3579, -3.1117) (23.0997, -3.0023) knots 0 0 0 1 2 2 2
  spline S23 degree 2 poles (23.0997, -3.0023) (22.8503, -3.1292) (22.7453, -3.2342) knots 0 0 0 1 1 1
  spline S24 degree 2 poles (22.7453, -3.2342) (22.6052, -3.383) (22.4696, -3.79) (22.4696, -4.1751) knots 0 0 0 1 2 2 2
  line L28 (22.4696, -4.1751) -> (22.4696, -5.3129)
  line L29 (22.4696, -5.3129) -> (22.7671, -4.9234)
  line L30 (22.7671, -4.9234) -> (23.5592, -4.9234)
  spline S25 degree 2 poles (22.4433, -3.383) (22.1326, -3.6237) (21.9488, -4.0657) (21.9488, -4.6171) knots 0 0 0 1 2 2 2
  line L31 (21.9488, -4.6171) -> (21.9488, -6.652)
  spline S26 degree 2 poles (21.9488, -6.652) (21.9488, -7.1509) (21.695, -7.5535) (21.3274, -7.7023) knots 0 0 0 1 2 2 2
  spline S27 degree 2 poles (21.3274, -7.7023) (21.4893, -7.711) (21.6031, -7.711) knots 0 0 0 1 1 1
  spline S28 degree 2 poles (21.6031, -7.711) (21.8657, -7.711) (22.1982, -7.5272) (22.3033, -7.2603) (22.3033, -6.9189) knots 0 0 0 1 2 3 3 3
  line L32 (22.3033, -6.9189) -> (22.3033, -4.2101)
  spline S29 degree 2 poles (22.3033, -4.2101) (22.3033, -3.9037) (22.3427, -3.6981) knots 0 0 0 1 1 1
  spline S30 degree 2 poles (22.3427, -3.6981) (22.3645, -3.5712) (22.4433, -3.383) knots 0 0 0 1 1 1
  line L33 (24.8852, -5.4617) -> (24.2901, -5.4617)
  line L34 (24.2901, -5.4617) -> (24.2901, -6.3938)
  spline S31 degree 2 poles (24.2901, -6.3938) (24.2901, -6.8752) (24.3557, -7.0108) knots 0 0 0 1 1 1
  spline S32 degree 2 poles (24.3557, -7.0108) (24.4607, -7.2471) (24.6358, -7.2471) knots 0 0 0 1 1 1
  spline S33 degree 2 poles (24.6358, -7.2471) (24.7277, -7.2471) (24.8852, -7.1071) knots 0 0 0 1 1 1
  line L35 (24.8852, -7.1071) -> (24.8852, -5.4617)
  line L36 (24.8852, -3.2473) -> (24.2901, -3.6368)
  line L37 (24.2901, -3.6368) -> (24.2901, -4.9234)
  line L38 (24.2901, -4.9234) -> (24.8852, -4.9234)
  line L39 (24.8852, -4.9234) -> (24.8852, -3.2473)
  line L40 (30.2591, -4.6696) -> (30.2591, -7.3565)
  spline S34 degree 2 poles (30.2591, -7.3565) (29.7165, -7.5754) (29.4758, -7.7154) knots 0 0 0 1 1 1
  spline S35 degree 2 poles (29.4758, -7.7154) (29.292, -7.8204) (29.1257, -7.9736) knots 0 0 0 1 1 1
  spline S36 degree 2 poles (29.1257, -7.9736) (28.605, -7.6585) (28.2636, -7.536) knots 0 0 0 1 1 1
  spline S37 degree 2 poles (28.2636, -7.536) (28.0054, -7.4441) (27.6772, -7.4309) knots 0 0 0 1 1 1
  line L41 (27.6772, -7.4309) -> (27.6422, -7.3609)
  spline S38 degree 2 poles (27.6422, -7.3609) (27.7779, -7.2471) (27.8129, -7.1509) knots 0 0 0 1 1 1
  spline S39 degree 2 poles (27.8129, -7.1509) (27.8654, -7.0283) (27.8654, -6.7395) knots 0 0 0 1 1 1
  line L42 (27.8654, -6.7395) -> (27.8654, -4.7615)
  spline S40 degree 2 poles (27.8654, -4.7615) (28.5262, -4.5427) (28.9944, -4.1444) knots 0 0 0 1 1 1
  spline S41 degree 2 poles (28.9944, -4.1444) (29.5021, -4.4814) (30.2591, -4.6696) knots 0 0 0 1 1 1
  line L43 (28.5918, -7.0065) -> (29.5283, -7.3916)
  line L44 (29.5283, -7.3916) -> (29.5283, -5.1116)
  spline S42 degree 2 poles (29.5283, -5.1116) (29.0863, -4.9015) (28.9025, -4.8359) knots 0 0 0 1 1 1
  spline S43 degree 2 poles (28.9025, -4.8359) (28.7756, -4.7921) (28.5918, -4.7571) knots 0 0 0 1 1 1
  line L45 (28.5918, -4.7571) -> (28.5918, -7.0065)
  line L46 (33.1999, -4.1444) -> (33.6901, -4.6827)
  line L47 (33.6901, -4.6827) -> (34.0402, -4.3457)
  line L48 (34.0402, -4.3457) -> (34.1364, -4.442)
  spline S44 degree 2 poles (34.1364, -4.442) (33.887, -4.674) (33.8301, -4.7921) knots 0 0 0 1 1 1
  spline S45 degree 2 poles (33.8301, -4.7921) (33.7601, -4.9497) (33.7601, -5.2297) knots 0 0 0 1 1 1
  line L49 (33.7601, -5.2297) -> (33.7601, -6.9408)
  spline S46 degree 2 poles (33.7601, -6.9408) (33.7601, -7.1771) (33.8345, -7.2953) knots 0 0 0 1 1 1
  spline S47 degree 2 poles (33.8345, -7.2953) (33.8826, -7.3697) (33.9395, -7.3697) knots 0 0 0 1 1 1
  spline S48 degree 2 poles (33.9395, -7.3697) (33.992, -7.3697) (34.1802, -7.234) knots 0 0 0 1 1 1
  line L50 (34.1802, -7.234) -> (34.2633, -7.3434)
  line L51 (34.2633, -7.3434) -> (33.4975, -7.9736)
  spline S49 degree 2 poles (33.4975, -7.9736) (33.1999, -7.7504) (33.0293, -7.4047) (33.0293, -7.0152) knots 0 0 0 1 2 2 2
  line L52 (33.0293, -7.0152) -> (33.0293, -5.0503)
  line L53 (33.0293, -5.0503) -> (32.7098, -4.7177)
  line L54 (32.7098, -4.7177) -> (32.0971, -5.2078)
  line L55 (32.0971, -5.2078) -> (32.0971, -7.199)
  line L56 (32.0971, -7.199) -> (32.3685, -7.4572)
  line L57 (32.3685, -7.4572) -> (31.7339, -7.9736)
  line L58 (31.7339, -7.9736) -> (31.095, -7.4572)
  line L59 (31.095, -7.4572) -> (31.3663, -7.199)
  line L60 (31.3663, -7.199) -> (31.3663, -5.3698)
  spline S50 degree 2 poles (31.3663, -5.3698) (31.3663, -4.9759) (31.2875, -4.8402) knots 0 0 0 1 1 1
  spline S51 degree 2 poles (31.2875, -4.8402) (31.235, -4.7483) (31.165, -4.7483) knots 0 0 0 1 1 1
  spline S52 degree 2 poles (31.165, -4.7483) (31.0906, -4.7483) (30.9506, -4.884) knots 0 0 0 1 1 1
  line L61 (30.9506, -4.884) -> (30.8631, -4.7746)
  line L62 (30.8631, -4.7746) -> (31.6245, -4.1444)
  spline S53 degree 2 poles (31.6245, -4.1444) (31.9396, -4.3808) (32.0971, -4.6564) (32.0971, -4.8971) knots 0 0 0 1 2 2 2
  line L63 (32.0971, -4.8971) -> (32.0971, -5.0284)
  line L64 (32.0971, -5.0284) -> (33.1999, -4.1444)
  line L65 (35.3836, -4.1444) -> (36.0182, -4.6696)
  line L66 (36.0182, -4.6696) -> (35.7337, -4.9497)
  line L67 (35.7337, -4.9497) -> (35.7337, -6.9058)
  spline S54 degree 2 poles (35.7337, -6.9058) (35.7337, -7.2121) (35.8388, -7.4003) (35.8913, -7.4003) knots 0 0 0 1 2 2 2
  spline S55 degree 2 poles (35.8913, -7.4003) (35.9307, -7.4003) (35.9657, -7.3828) knots 0 0 0 1 1 1
  spline S56 degree 2 poles (35.9657, -7.3828) (36.0094, -7.3565) (36.1538, -7.234) knots 0 0 0 1 1 1
  line L68 (36.1538, -7.234) -> (36.237, -7.3434)
  line L69 (36.237, -7.3434) -> (35.4712, -7.9736)
  spline S57 degree 2 poles (35.4712, -7.9736) (35.1823, -7.7679) (35.016, -7.4047) (35.016, -6.9539) knots 0 0 0 1 2 2 2
  line L70 (35.016, -6.9539) -> (35.016, -4.9497)
  line L71 (35.016, -4.9497) -> (34.7447, -4.6696)
  line L72 (34.7447, -4.6696) -> (35.3836, -4.1444)
  line L73 (35.6506, -2.9191) -> (36.1057, -2.9191)
  line L74 (36.1057, -2.9191) -> (35.6112, -3.6937)
  line L75 (35.6112, -3.6937) -> (35.4668, -3.6937)
  line L76 (35.4668, -3.6937) -> (35.6506, -2.9191)
  line L77 (37.9262, -4.1444) -> (38.8583, -4.674)
  line L78 (38.8583, -4.674) -> (38.482, -5.2385)
  line L79 (38.482, -5.2385) -> (37.773, -4.8315)
  line L80 (37.773, -4.8315) -> (37.773, -7.1246)
  line L81 (37.773, -7.1246) -> (38.4776, -7.4397)
  line L82 (38.4776, -7.4397) -> (38.8539, -7.1596)
  line L83 (38.8539, -7.1596) -> (38.8933, -7.3172)
  line L84 (38.8933, -7.3172) -> (38.005, -7.9736)
  spline S58 degree 2 poles (38.005, -7.9736) (37.6592, -7.781) (37.1735, -7.5972) (36.819, -7.5272) knots 0 0 0 1 2 2 2
  line L85 (36.819, -7.5272) -> (36.819, -7.4397)
  spline S59 degree 2 poles (36.819, -7.4397) (36.9459, -7.3522) (36.9853, -7.2515) knots 0 0 0 1 1 1
  spline S60 degree 2 poles (36.9853, -7.2515) (37.0422, -7.1115) (37.0422, -6.8139) knots 0 0 0 1 1 1
  line L86 (37.0422, -6.8139) -> (37.0422, -4.7746)
  spline S61 degree 2 poles (37.0422, -4.7746) (37.4886, -4.5689) (37.9262, -4.1444) knots 0 0 0 1 1 1
  line L87 (41.7728, -4.2976) -> (41.9041, -4.3457)
  spline S62 degree 2 poles (41.9041, -4.3457) (41.7072, -4.6477) (41.6022, -4.9672) (41.6022, -5.2429) knots 0 0 0 1 2 2 2
  line L88 (41.6022, -5.2429) -> (41.6022, -6.7701)
  spline S63 degree 2 poles (41.6022, -6.7701) (41.6022, -7.1509) (41.7116, -7.3434) (41.786, -7.3434) knots 0 0 0 1 2 2 2
  spline S64 degree 2 poles (41.786, -7.3434) (41.8254, -7.3434) (41.8647, -7.3215) knots 0 0 0 1 1 1
  spline S65 degree 2 poles (41.8647, -7.3215) (41.891, -7.3084) (42.0223, -7.2034) knots 0 0 0 1 1 1
  line L89 (42.0223, -7.2034) -> (42.1054, -7.3128)
  line L90 (42.1054, -7.3128) -> (41.3484, -7.9736)
  spline S66 degree 2 poles (41.3484, -7.9736) (41.0683, -7.7592) (40.8801, -7.4178) (40.8713, -7.1115) knots 0 0 0 1 2 2 2
  line L91 (40.8713, -7.1115) -> (39.7817, -7.9736)
  spline S67 degree 2 poles (39.7817, -7.9736) (39.1646, -7.4703) (39.1646, -6.9802) knots 0 0 0 1 1 1
  spline S68 degree 2 poles (39.1646, -6.9802) (39.1646, -6.652) (39.2959, -6.3632) knots 0 0 0 1 1 1
  spline S69 degree 2 poles (39.2959, -6.3632) (39.4754, -5.9868) (39.9086, -5.4835) knots 0 0 0 1 1 1
  line L92 (39.9086, -5.4835) -> (39.471, -4.5646)
  line L93 (39.471, -4.5646) -> (39.5235, -4.4683)
  spline S70 degree 2 poles (39.5235, -4.4683) (39.6635, -4.477) (39.7335, -4.477) knots 0 0 0 1 1 1
  spline S71 degree 2 poles (39.7335, -4.477) (40.1537, -4.477) (40.4775, -4.1444) knots 0 0 0 1 1 1
  spline S72 degree 2 poles (40.4775, -4.1444) (40.7401, -4.2976) (41.3615, -4.4814) (41.5234, -4.4814) knots 0 0 0 1 2 2 2
  spline S73 degree 2 poles (41.5234, -4.4814) (41.6022, -4.4814) (41.6809, -4.4289) (41.7728, -4.2976) knots 0 0 0 1 2 2 2
  line L94 (40.8713, -6.0524) -> (40.0005, -5.6411)
  spline S74 degree 2 poles (40.0005, -5.6411) (39.7992, -6.0831) (39.7992, -6.4113) knots 0 0 0 1 1 1
  spline S75 degree 2 poles (39.7992, -6.4113) (39.7992, -6.9933) (40.3243, -7.3697) knots 0 0 0 1 1 1
  line L95 (40.3243, -7.3697) -> (40.8713, -6.9364)
  line L96 (40.8713, -6.9364) -> (40.8713, -6.0524)
  line L97 (40.8713, -4.9803) -> (39.6416, -4.6039)
  line L98 (39.6416, -4.6039) -> (40.0793, -5.5317)
  line L99 (40.0793, -5.5317) -> (40.8713, -5.9037)
  line L100 (40.8713, -5.9037) -> (40.8713, -4.9803)
  line L101 (47.7113, -2.534) -> (47.847, -2.6128)
  spline S76 degree 2 poles (47.847, -2.6128) (47.545, -3.1248) (47.2912, -3.9081) (47.2518, -4.4333) knots 0 0 0 1 2 2 2
  line L102 (47.2518, -4.4333) -> (48.6303, -3.3436)
  line L103 (48.6303, -3.3436) -> (49.4661, -4.3151)
  line L104 (49.4661, -4.3151) -> (48.0351, -5.3304)
  spline S77 degree 2 poles (48.0351, -5.3304) (48.3633, -5.5098) (48.8579, -6.0306) (49.5099, -7.1377) (49.6543, -7.2909) (49.72, -7.2909) knots 0 0 0 1 2 3 4 4 4
  spline S78 degree 2 poles (49.72, -7.2909) (49.79, -7.2909) (49.93, -7.1509) knots 0 0 0 1 1 1
  line L105 (49.93, -7.1509) -> (50.1182, -6.9758)
  line L106 (50.1182, -6.9758) -> (50.2276, -7.1071)
  line L107 (50.2276, -7.1071) -> (49.3349, -7.9736)
  spline S79 degree 2 poles (49.3349, -7.9736) (49.1467, -7.8423) (48.9322, -7.5666) (48.569, -6.9146) knots 0 0 0 1 2 2 2
  line L108 (48.569, -6.9146) -> (47.6413, -7.9736)
  spline S80 degree 2 poles (47.6413, -7.9736) (47.2124, -7.7854) (46.5166, -7.6191) (46.149, -7.6191) knots 0 0 0 1 2 2 2
  spline S81 degree 2 poles (46.149, -7.6191) (45.7902, -7.6191) (45.1031, -7.781) (44.6567, -7.9736) knots 0 0 0 1 2 2 2
  line L109 (44.6567, -7.9736) -> (44.5386, -7.8073)
  spline S82 degree 2 poles (44.5386, -7.8073) (45.2431, -7.2471) (45.5495, -6.8139) knots 0 0 0 1 1 1
  spline S83 degree 2 poles (45.5495, -6.8139) (45.6983, -6.5995) (45.6983, -6.3982) knots 0 0 0 1 1 1
  spline S84 degree 2 poles (45.6983, -6.3982) (45.6983, -6.2056) (45.4444, -5.9562) (45.2738, -5.9562) knots 0 0 0 1 2 2 2
  spline S85 degree 2 poles (45.2738, -5.9562) (45.1162, -5.9562) (44.9937, -6.1137) knots 0 0 0 1 1 1
  line L110 (44.9937, -6.1137) -> (44.8668, -6.0524)
  spline S86 degree 2 poles (44.8668, -6.0524) (44.9324, -5.8424) (45.2388, -5.6105) (45.4313, -5.6105) knots 0 0 0 1 2 2 2
  spline S87 degree 2 poles (45.4313, -5.6105) (45.5582, -5.6105) (45.8295, -5.7111) (45.9783, -5.8161) knots 0 0 0 1 2 2 2
  spline S88 degree 2 poles (45.9783, -5.8161) (45.9871, -5.698) (45.9871, -5.6148) knots 0 0 0 1 1 1
  spline S89 degree 2 poles (45.9871, -5.6148) (45.9871, -5.2297) (45.5407, -4.7571) (45.23, -4.7571) knots 0 0 0 1 2 2 2
  spline S90 degree 2 poles (45.23, -4.7571) (45.0506, -4.7571) (44.8712, -4.9146) knots 0 0 0 1 1 1
  line L111 (44.8712, -4.9146) -> (44.7486, -4.8665)
  spline S91 degree 2 poles (44.7486, -4.8665) (44.8362, -4.6389) (45.1731, -4.407) (45.3963, -4.407) knots 0 0 0 1 2 2 2
  spline S92 degree 2 poles (45.3963, -4.407) (45.5145, -4.407) (45.7945, -4.5033) (45.9477, -4.5996) knots 0 0 0 1 2 2 2
  spline S93 degree 2 poles (45.9477, -4.5996) (45.9389, -4.4508) (45.9389, -4.337) knots 0 0 0 1 1 1
  spline S94 degree 2 poles (45.9389, -4.337) (45.9389, -4.0044) (46.2146, -3.4968) (46.8579, -2.8228) knots 0 0 0 1 2 2 2
  spline S95 degree 2 poles (46.8579, -2.8228) (46.4772, -3.0416) (46.0352, -3.1904) (45.8164, -3.1904) knots 0 0 0 1 2 2 2
  spline S96 degree 2 poles (45.8164, -3.1904) (45.7026, -3.1904) (45.335, -3.1248) (45.2563, -3.1248) knots 0 0 0 1 2 2 2
  spline S97 degree 2 poles (45.2563, -3.1248) (44.9937, -3.1248) (44.6305, -3.3917) (44.4686, -3.7068) knots 0 0 0 1 2 2 2
  line L112 (44.4686, -3.7068) -> (44.346, -3.6806)
  spline S98 degree 2 poles (44.346, -3.6806) (44.4204, -3.3173) (44.5298, -3.1379) knots 0 0 0 1 1 1
  spline S99 degree 2 poles (44.5298, -3.1379) (44.7005, -2.8491) (45.2038, -2.534) (45.4663, -2.534) knots 0 0 0 1 2 2 2
  spline S100 degree 2 poles (45.4663, -2.534) (45.6676, -2.534) (46.2628, -2.7222) (46.4553, -2.7222) knots 0 0 0 1 2 2 2
  spline S101 degree 2 poles (46.4553, -2.7222) (46.766, -2.7222) (47.1293, -2.534) knots 0 0 0 1 1 1
  line L113 (47.1293, -2.534) -> (47.2562, -2.6128)
  spline S102 degree 2 poles (47.2562, -2.6128) (46.9586, -3.046) (46.661, -4.1576) (46.661, -4.6783) knots 0 0 0 1 2 2 2
  line L114 (46.661, -4.6783) -> (46.6741, -5.7024)
  spline S103 degree 2 poles (46.6741, -5.7024) (46.6741, -5.9299) (46.5297, -6.315) (46.2628, -6.6213) (46.2278, -6.6476) knots 0 0 0 1 2 3 3 3
  line L115 (46.2278, -6.6476) -> (45.1731, -7.5316)
  spline S104 degree 2 poles (45.1731, -7.5316) (45.4532, -7.3828) (45.7683, -7.2471) knots 0 0 0 1 1 1
  spline S105 degree 2 poles (45.7683, -7.2471) (46.3416, -7.0021) (46.8317, -6.6432) (47.0986, -6.0875) (47.0986, -5.663) knots 0 0 0 1 2 3 3 3
  line L116 (47.0986, -5.663) -> (47.0855, -4.5427)
  spline S106 degree 2 poles (47.0855, -4.5427) (47.0855, -4.1401) (47.3656, -3.1029) (47.7113, -2.534) knots 0 0 0 1 2 2 2
  spline S107 degree 2 poles (48.4859, -6.7745) (48.1533, -6.2406) (47.5888, -5.8424) (47.2518, -5.8293) knots 0 0 0 1 2 2 2
  spline S108 degree 2 poles (47.2518, -5.8293) (47.243, -6.2362) (46.9411, -6.7745) (46.591, -7.0196) knots 0 0 0 1 2 2 2
  spline S109 degree 2 poles (46.591, -7.0196) (47.1424, -7.0502) (47.6675, -7.1771) (47.987, -7.3434) knots 0 0 0 1 2 2 2
  line L117 (47.987, -7.3434) -> (48.4859, -6.7745)
  line L118 (48.162, -3.9169) -> (47.2518, -4.6433)
  line L119 (47.2518, -4.6433) -> (47.2518, -4.7527)
  line L120 (47.2518, -4.7527) -> (47.2606, -5.3216)
  line L121 (47.2606, -5.3216) -> (47.2518, -5.6717)
  line L122 (47.2518, -5.6717) -> (48.7616, -4.6083)
  line L123 (48.7616, -4.6083) -> (48.162, -3.9169)
  line L124 (52.5863, -4.1444) -> (53.1246, -4.7921)
  line L125 (53.1246, -4.7921) -> (52.5863, -5.2735)
  line L126 (52.5863, -5.2735) -> (52.1312, -4.7046)
  line L127 (52.1312, -4.7046) -> (51.7768, -5.0284)
  line L128 (51.7768, -5.0284) -> (51.7768, -7.1202)
  line L129 (51.7768, -7.1202) -> (52.1881, -7.4134)
  line L130 (52.1881, -7.4134) -> (52.5557, -7.129)
  line L131 (52.5557, -7.129) -> (52.6389, -7.2384)
  line L132 (52.6389, -7.2384) -> (51.7199, -7.9736)
  spline S110 degree 2 poles (51.7199, -7.9736) (51.4267, -7.711) (51.0284, -7.4835) (50.7921, -7.4178) knots 0 0 0 1 2 2 2
  line L133 (50.7921, -7.4178) -> (50.7921, -7.339)
  spline S111 degree 2 poles (50.7921, -7.339) (50.9497, -7.2296) (51.0459, -7.0021) (51.0459, -6.6826) knots 0 0 0 1 2 2 2
  line L134 (51.0459, -6.6826) -> (51.0459, -5.2122)
  spline S112 degree 2 poles (51.0459, -5.2122) (51.0459, -4.9365) (50.9234, -4.7527) (50.849, -4.7527) knots 0 0 0 1 2 2 2
  spline S113 degree 2 poles (50.849, -4.7527) (50.7702, -4.7527) (50.6302, -4.9015) knots 0 0 0 1 1 1
  line L135 (50.6302, -4.9015) -> (50.5427, -4.7921)
  line L136 (50.5427, -4.7921) -> (51.291, -4.1444)
  spline S114 degree 2 poles (51.291, -4.1444) (51.593, -4.3764) (51.7067, -4.5514) knots 0 0 0 1 1 1
  spline S115 degree 2 poles (51.7067, -4.5514) (51.7768, -4.6564) (51.7768, -4.849) knots 0 0 0 1 1 1
  line L137 (51.7768, -4.849) -> (52.5863, -4.1444)
  line L138 (56.061, -4.2976) -> (56.1923, -4.3457)
  spline S116 degree 2 poles (56.1923, -4.3457) (55.9954, -4.6477) (55.8904, -4.9672) (55.8904, -5.2429) knots 0 0 0 1 2 2 2
  line L139 (55.8904, -5.2429) -> (55.8904, -6.7701)
  spline S117 degree 2 poles (55.8904, -6.7701) (55.8904, -7.1509) (55.9998, -7.3434) (56.0742, -7.3434) knots 0 0 0 1 2 2 2
  spline S118 degree 2 poles (56.0742, -7.3434) (56.1135, -7.3434) (56.1529, -7.3215) knots 0 0 0 1 1 1
  spline S119 degree 2 poles (56.1529, -7.3215) (56.1792, -7.3084) (56.3105, -7.2034) knots 0 0 0 1 1 1
  line L140 (56.3105, -7.2034) -> (56.3936, -7.3128)
  line L141 (56.3936, -7.3128) -> (55.6365, -7.9736)
  spline S120 degree 2 poles (55.6365, -7.9736) (55.3565, -7.7592) (55.1683, -7.4178) (55.1595, -7.1115) knots 0 0 0 1 2 2 2
  line L142 (55.1595, -7.1115) -> (54.0699, -7.9736)
  spline S121 degree 2 poles (54.0699, -7.9736) (53.4528, -7.4703) (53.4528, -6.9802) knots 0 0 0 1 1 1
  spline S122 degree 2 poles (53.4528, -6.9802) (53.4528, -6.652) (53.5841, -6.3632) knots 0 0 0 1 1 1
  spline S123 degree 2 poles (53.5841, -6.3632) (53.7635, -5.9868) (54.1968, -5.4835) knots 0 0 0 1 1 1
  line L143 (54.1968, -5.4835) -> (53.7592, -4.5646)
  line L144 (53.7592, -4.5646) -> (53.8117, -4.4683)
  spline S124 degree 2 poles (53.8117, -4.4683) (53.9517, -4.477) (54.0217, -4.477) knots 0 0 0 1 1 1
  spline S125 degree 2 poles (54.0217, -4.477) (54.4418, -4.477) (54.7657, -4.1444) knots 0 0 0 1 1 1
  spline S126 degree 2 poles (54.7657, -4.1444) (55.0282, -4.2976) (55.6497, -4.4814) (55.8116, -4.4814) knots 0 0 0 1 2 2 2
  spline S127 degree 2 poles (55.8116, -4.4814) (55.8904, -4.4814) (55.9691, -4.4289) (56.061, -4.2976) knots 0 0 0 1 2 2 2
  line L145 (55.1595, -6.0524) -> (54.2887, -5.6411)
  spline S128 degree 2 poles (54.2887, -5.6411) (54.0874, -6.0831) (54.0874, -6.4113) knots 0 0 0 1 1 1
  spline S129 degree 2 poles (54.0874, -6.4113) (54.0874, -6.9933) (54.6125, -7.3697) knots 0 0 0 1 1 1
  line L146 (54.6125, -7.3697) -> (55.1595, -6.9364)
  line L147 (55.1595, -6.9364) -> (55.1595, -6.0524)
  line L148 (55.1595, -4.9803) -> (53.9298, -4.6039)
  line L149 (53.9298, -4.6039) -> (54.3674, -5.5317)
  line L150 (54.3674, -5.5317) -> (55.1595, -5.9037)
  line L151 (55.1595, -5.9037) -> (55.1595, -4.9803)
  line L152 (58.4985, -2.9979) -> (58.3891, -3.593)
  line L153 (58.3891, -3.593) -> (57.7327, -3.4443)
  line L154 (57.7327, -3.4443) -> (57.7327, -4.3107)
  line L155 (57.7327, -4.3107) -> (58.2885, -4.3107)
  line L156 (58.2885, -4.3107) -> (58.2885, -4.7133)
  line L157 (58.2885, -4.7133) -> (57.7327, -4.7133)
  line L158 (57.7327, -4.7133) -> (57.7327, -7.1202)
  line L159 (57.7327, -7.1202) -> (58.1397, -7.4266)
  line L160 (58.1397, -7.4266) -> (58.4198, -7.2034)
  line L161 (58.4198, -7.2034) -> (58.5029, -7.304)
  line L162 (58.5029, -7.304) -> (57.6715, -7.9736)